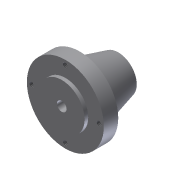
# Autodesk Inventor part: wheel_hub
Saved by Autodesk Inventor 2012 (Build 160160000, 160)
## iProperties
Created: 2012-04-25
Part Number: wheel_hub
Material: Default
Document SubType Name: Modeling
Designer: Antonella Wilby
Density: 1 g/cm^3
Author: Antonella Wilby
Autodesk Inventor part; units mm, degrees
ref_plane "YZ Plane" through (0, 0, 0) normal (1, 0, 0) x (0, 1, 0)
ref_plane "XZ Plane" through (0, 0, 0) normal (0, 1, 0) x (-1, 0, 0)
ref_plane "XY Plane" through (0, 0, 0) normal (0, 0, 1) x (1, 0, 0)
sketch "Sketch1" plane through (0, 0, 0) normal (0, 0, 1) x (1, 0, 0)
  line L0 (-71.12, 0) -> (71.12, 0) projected
  line L1 (0, -71.12) -> (0, 71.12) projected
  circle A0 centre (0, 0) radius 50.8
  dimension "d0" = 101.6
  constraints: 1 centre point, 1 coincident
  measures "d0" diameter of A0
extrude "Extrusion1" add sketch "Sketch1" against normal blind 19.05
sketch "Sketch2" plane through (0, 0, 0) normal (0, 0, 1) x (1, 0, 0)
  circle A0 centre (0, 0) radius 50.8 projected
  circle A1 centre (0, 0) radius 30.1625
  dimension "d3" = 60.325
  constraints: 1 centre point, 1 coincident
  measures "d3" diameter of A1
extrude "Extrusion2" add sketch "Sketch2" along normal blind 4.7625 contours A1
sketch "Sketch3" plane through (0, 0, 0) normal (0, 0, 1) x (1, 0, 0)
  circle A0 centre (0, 0) radius 30.1625 projected
  point P0 (0, 44.45)
  point P1 (-44.45, 0)
  point P2 (0, -44.45)
  point P3 (44.45, 0)
  dimension "d8" = 360
  dimension "d35" = 88.9
  constraints: 5 other
  measures "d35" distance of point (44.45, 0) point (-44.45, 0)
hole "Hole1" at (0, 44.45, 0) at (-44.45, 0, 0) at (0, -44.45, 0) at (44.45, 0, 0) direction (0, 0, -1) diameter 6.4008 end through all thread size "5/16-18 UNC" class "2B" standard "ANSI Unified Screw Threads"
sketch "Sketch5" plane through (0, 0, -19.05) normal (0, 0, -1) x (-1, 0, 0)
  circle A0 centre (0, 0) radius 50.8 projected
  circle A1 centre (0, 0) radius 38.1
  dimension "d17" = 76.2
  constraints: 1 centre point, 1 coincident
  measures "d17" diameter of A1
extrude "Extrusion3" add sketch "Sketch5" along normal blind 50.8 draft -15 contours A1
sketch "Sketch6" plane through (0, 0, -69.85) normal (0, 0, -1) x (-1, 0, 0)
  circle A0 centre (0, 0) radius 24.4882 projected
  point P0 (0, 17.4625)
  point P1 (-15.123, 8.7313)
  point P2 (-15.123, -8.7312)
  point P3 (0, -17.4625)
  point P4 (15.123, -8.7313)
  point P5 (15.123, 8.7312)
  dimension "d22" = 360
  dimension "d24" = 17.4625
  constraints: 7 other
  measures "d24" distance of point (0, 17.463) A0.centre
hole "Hole2" at (0, 17.4625, -69.85) at (15.123, 8.7313, -69.85) at (15.123, -8.7312, -69.85) at (0, -17.4625, -69.85) at (-15.123, -8.7313, -69.85) at (-15.123, 8.7312, -69.85) direction (0, 0, 1) diameter 3.683 depth 12.7 tip angle 118 thread size "10-24 UNC" class "2B" standard "ANSI Unified Screw Threads"
sketch "Sketch7" plane through (0, 0, 4.7625) normal (0, 0, 1) x (1, 0, 0)
  circle A0 centre (0, 0) radius 30.1625 projected
  circle A1 centre (0, 0) radius 6.35
  dimension "d32" = 12.7
  constraints: 1 centre point, 1 coincident
  measures "d32" diameter of A1
extrude "Extrusion4" cut sketch "Sketch7" against normal through all contours A1
body "Solid1"
